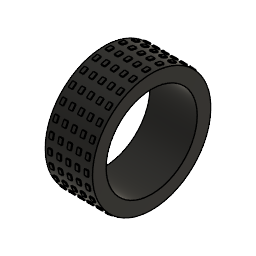
Wheel (Autodesk Fusion 360 archive; units mm, degrees)
design "Piece1"
part number: 2026-01-02-17-32-33-546
Autodesk Fusion 360 part; units mm, degrees
note: some values were not read from the file. Chosen so that the rebuilt part matches the saved one: which bodies a step acts on.
sketch "Boceto1" plane through (0, 0, 0) normal (1, 0, 0) x (0, 1, 0)
  circle A0 centre (0, 0) radius 25
  circle A1 centre (0, 0) radius 32.5
  dimension "d1" = 50
  dimension "d2" = 65
  constraint coincident A0.centre A1.centre
  constraint concentric A0 A1
  measures "d1" diameter of A0
  measures "d2" diameter of A1
extrude "Ancho" add sketch "Boceto1" along normal blind 26 makes body 1
ref_plane "PlanoDeObra1" through (16.1353, 0, 32.5) normal (0, 0, 1) x (0, 1, 0)
sketch "Boceto2" plane through (0, 0, 32.5) normal (0, 0, 1) x (1, 0, 0)
  line L0 (0, 0) -> (13, 0) construction
  line L1 (14, 1.5) -> (12, 1.5)
  line L2 (12, 1.5) -> (12, -1.5)
  line L3 (12, -1.5) -> (14, -1.5)
  line L4 (14, -1.5) -> (14, 1.5)
  line L5 (14, 1.5) -> (12, -1.5) construction
  line L6 (12, 1.5) -> (14, -1.5) construction
  line L7 (13, 0) -> (13, 32.5) construction
  line L8 (4, 1.5) -> (2, 1.5)
  line L9 (2, 1.5) -> (2, -1.5)
  line L10 (4, -1.5) -> (4, 1.5)
  line L11 (2, -1.5) -> (4, -1.5)
  line L12 (9, 1.5) -> (7, 1.5)
  line L13 (7, 1.5) -> (7, -1.5)
  line L14 (9, -1.5) -> (9, 1.5)
  line L15 (7, -1.5) -> (9, -1.5)
  line L16 (19, 1.5) -> (17, 1.5)
  line L17 (17, 1.5) -> (17, -1.5)
  line L18 (19, -1.5) -> (19, 1.5)
  line L19 (17, -1.5) -> (19, -1.5)
  line L20 (24, 1.5) -> (22, 1.5)
  line L21 (22, 1.5) -> (22, -1.5)
  line L22 (24, -1.5) -> (24, 1.5)
  line L23 (22, -1.5) -> (24, -1.5)
  point P0 (13, 0)
  dimension "d6" = 13
  dimension "d7" = 3
  dimension "d8" = 2
  dimension "d9" = 32.5
  dimension "d12" = 10
  dimension "d13" = 0
  constraint coincident L0.start origin
  constraint horizontal L0
  constraint horizontal L1
  constraint perpendicular L1 L2
  constraint parallel L1 L3
  constraint parallel L2 L4
  constraint coincident L5 P0
  constraint coincident L6 P0
  constraint coincident P0 L0.end
  constraint perpendicular L0 L7
  measures "d6" distance of L0.start P0
  measures "d7" distance of L1.end L2.end
  measures "d8" distance of L1.start L1.end
  measures "d9" distance of P0 L7.end
extrude "Altura" add sketch "Boceto2" along normal blind 0.5 separate body makes body 2 at (12.6667, -0.5, 32.5) makes body 3 at (7.6667, -0.5, 32.5) makes body 4 at (18.3333, -0.5, 32.5) makes body 5 at (2.6667, -0.5, 32.5) makes body 6 at (22.6667, -0.5, 32.5)
pattern_circular "Patrón C1" count 28 over 360 about axis through (0, 0, 0) along (1, 0, 0) of bodies 5 3 2 4 6 makes body 7 at (12.6667, -7.7194, 31.5739) makes body 8 at (12.6667, -14.5517, 29.0645) makes body 9 at (12.6667, -20.6543, 25.0978) makes body 10 at (12.6667, -25.7213, 19.8725) makes body 11 at (12.6667, -29.4984, 13.6507) makes body 12 at (12.6667, -31.7964, 6.7445) makes body 13 at (12.6667, -32.5, -0.5) makes body 14 at (12.6667, -31.5739, -7.7194) makes body 15 at (12.6667, -29.0645, -14.5517) makes body 16 at (12.6667, -25.0978, -20.6543) makes body 17 at (12.6667, -19.8725, -25.7213) makes body 18 at (12.6667, -13.6507, -29.4984) makes body 19 at (12.6667, -6.7445, -31.7964) makes body 20 at (12.6667, 0.5, -32.5) makes body 21 at (12.6667, 7.7194, -31.5739) makes body 22 at (12.6667, 14.5517, -29.0645) makes body 23 at (12.6667, 20.6543, -25.0978) makes body 24 at (12.6667, 25.7213, -19.8725) makes body 25 at (12.6667, 29.4984, -13.6507) makes body 26 at (12.6667, 31.7964, -6.7445) makes body 27 at (12.6667, 32.5, 0.5) makes body 28 at (12.6667, 31.5739, 7.7194) makes body 29 at (12.6667, 29.0645, 14.5517) makes body 30 at (12.6667, 25.0978, 20.6543) makes body 31 at (12.6667, 19.8725, 25.7213) makes body 32 at (12.6667, 13.6507, 29.4984) makes body 33 at (12.6667, 6.7445, 31.7964) makes body 34 at (7.6667, -7.7194, 31.5739) makes body 35 at (7.6667, -14.5517, 29.0645) makes body 36 at (7.6667, -20.6543, 25.0978) makes body 37 at (7.6667, -25.7213, 19.8725) makes body 38 at (7.6667, -29.4984, 13.6507) makes body 39 at (7.6667, -31.7964, 6.7445) makes body 40 at (7.6667, -32.5, -0.5) makes body 41 at (7.6667, -31.5739, -7.7194) makes body 42 at (7.6667, -29.0645, -14.5517) makes body 43 at (7.6667, -25.0978, -20.6543) makes body 44 at (7.6667, -19.8725, -25.7213) makes body 45 at (7.6667, -13.6507, -29.4984) makes body 46 at (7.6667, -6.7445, -31.7964) makes body 47 at (7.6667, 0.5, -32.5) makes body 48 at (7.6667, 7.7194, -31.5739) makes body 49 at (7.6667, 14.5517, -29.0645) makes body 50 at (7.6667, 20.6543, -25.0978) makes body 51 at (7.6667, 25.7213, -19.8725) makes body 52 at (7.6667, 29.4984, -13.6507) makes body 53 at (7.6667, 31.7964, -6.7445) makes body 54 at (7.6667, 32.5, 0.5) makes body 55 at (7.6667, 31.5739, 7.7194) makes body 56 at (7.6667, 29.0645, 14.5517) makes body 57 at (7.6667, 25.0978, 20.6543) makes body 58 at (7.6667, 19.8725, 25.7213) makes body 59 at (7.6667, 13.6507, 29.4984) makes body 60 at (7.6667, 6.7445, 31.7964) makes body 61 at (18.3333, -7.7194, 31.5739) makes body 62 at (18.3333, -14.5517, 29.0645) makes body 63 at (18.3333, -20.6543, 25.0978) makes body 64 at (18.3333, -25.7213, 19.8725) makes body 65 at (18.3333, -29.4984, 13.6507) makes body 66 at (18.3333, -31.7964, 6.7445) makes body 67 at (18.3333, -32.5, -0.5) makes body 68 at (18.3333, -31.5739, -7.7194) makes body 69 at (18.3333, -29.0645, -14.5517) makes body 70 at (18.3333, -25.0978, -20.6543) makes body 71 at (18.3333, -19.8725, -25.7213) makes body 72 at (18.3333, -13.6507, -29.4984) makes body 73 at (18.3333, -6.7445, -31.7964) makes body 74 at (18.3333, 0.5, -32.5) makes body 75 at (18.3333, 7.7194, -31.5739) makes body 76 at (18.3333, 14.5517, -29.0645) makes body 77 at (18.3333, 20.6543, -25.0978) makes body 78 at (18.3333, 25.7213, -19.8725) makes body 79 at (18.3333, 29.4984, -13.6507) makes body 80 at (18.3333, 31.7964, -6.7445) makes body 81 at (18.3333, 32.5, 0.5) makes body 82 at (18.3333, 31.5739, 7.7194) makes body 83 at (18.3333, 29.0645, 14.5517) makes body 84 at (18.3333, 25.0978, 20.6543) makes body 85 at (18.3333, 19.8725, 25.7213) makes body 86 at (18.3333, 13.6507, 29.4984) makes body 87 at (18.3333, 6.7445, 31.7964) makes body 88 at (2.6667, -7.7194, 31.5739) makes body 89 at (2.6667, -14.5517, 29.0645) makes body 90 at (2.6667, -20.6543, 25.0978) makes body 91 at (2.6667, -25.7213, 19.8725) makes body 92 at (2.6667, -29.4984, 13.6507) makes body 93 at (2.6667, -31.7964, 6.7445) makes body 94 at (2.6667, -32.5, -0.5) makes body 95 at (2.6667, -31.5739, -7.7194) makes body 96 at (2.6667, -29.0645, -14.5517) makes body 97 at (2.6667, -25.0978, -20.6543) makes body 98 at (2.6667, -19.8725, -25.7213) makes body 99 at (2.6667, -13.6507, -29.4984) makes body 100 at (2.6667, -6.7445, -31.7964) makes body 101 at (2.6667, 0.5, -32.5) makes body 102 at (2.6667, 7.7194, -31.5739) makes body 103 at (2.6667, 14.5517, -29.0645) makes body 104 at (2.6667, 20.6543, -25.0978) makes body 105 at (2.6667, 25.7213, -19.8725) makes body 106 at (2.6667, 29.4984, -13.6507) makes body 107 at (2.6667, 31.7964, -6.7445) makes body 108 at (2.6667, 32.5, 0.5) makes body 109 at (2.6667, 31.5739, 7.7194) makes body 110 at (2.6667, 29.0645, 14.5517) makes body 111 at (2.6667, 25.0978, 20.6543) makes body 112 at (2.6667, 19.8725, 25.7213) makes body 113 at (2.6667, 13.6507, 29.4984) makes body 114 at (2.6667, 6.7445, 31.7964) makes body 115 at (22.6667, -7.7194, 31.5739) makes body 116 at (22.6667, -14.5517, 29.0645) makes body 117 at (22.6667, -20.6543, 25.0978) makes body 118 at (22.6667, -25.7213, 19.8725) makes body 119 at (22.6667, -29.4984, 13.6507) makes body 120 at (22.6667, -31.7964, 6.7445) makes body 121 at (22.6667, -32.5, -0.5) makes body 122 at (22.6667, -31.5739, -7.7194) makes body 123 at (22.6667, -29.0645, -14.5517) makes body 124 at (22.6667, -25.0978, -20.6543) makes body 125 at (22.6667, -19.8725, -25.7213) makes body 126 at (22.6667, -13.6507, -29.4984) makes body 127 at (22.6667, -6.7445, -31.7964) makes body 128 at (22.6667, 0.5, -32.5) makes body 129 at (22.6667, 7.7194, -31.5739) makes body 130 at (22.6667, 14.5517, -29.0645) makes body 131 at (22.6667, 20.6543, -25.0978) makes body 132 at (22.6667, 25.7213, -19.8725) makes body 133 at (22.6667, 29.4984, -13.6507) makes body 134 at (22.6667, 31.7964, -6.7445) makes body 135 at (22.6667, 32.5, 0.5) makes body 136 at (22.6667, 31.5739, 7.7194) makes body 137 at (22.6667, 29.0645, 14.5517) makes body 138 at (22.6667, 25.0978, 20.6543) makes body 139 at (22.6667, 19.8725, 25.7213) makes body 140 at (22.6667, 13.6507, 29.4984) makes body 141 at (22.6667, 6.7445, 31.7964)
combine "Combinar1" operation add target body 1 tool bodies 21 18 26 4 5 10 11 13 7 14 15 6 8 9 12 3 16 17 19 20 22 23 24 25 28 29 30 32 34 35 36 33 38 39 40 41 37 42 27 43 44 45 46 47 48 49 31 55 57 58 59 54 52 53 51 56 50 64 78 80 84 86 88 67 83 92 94 82 97 60 62 68 69 66 61 63 71 65 72 73 74 75 70 76 77 79 81 85 87 89 90 91 93 95 96 99 102 103 104 105 107 100 108 109 110 111 101 98 112 113 114 106 121 115 122 116 118 120 119 123 117 124 128 140 130 132 134 136 139 126 141 135 138 127 125 129 133 137 131 2
equation "d6 = ( 26 / 2 ) * 1 mm"
equation "d9 = ( 65 / 2 ) * 1 mm"
named bodies: "Llanta"

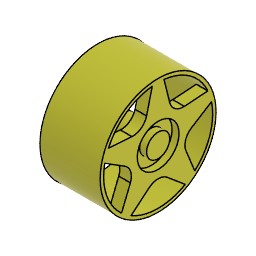
design "Piece2"
part number: 2026-01-02-23-41-02-488
Autodesk Fusion 360 part; units mm, degrees
sketch "Boceto1" plane through (0, 0, 0) normal (1, 0, 0) x (0, 1, 0)
  circle A0 centre (0, 0) radius 25
  dimension "d1" = 50
  constraint coincident A0.centre origin
  measures "d1" diameter of A0
extrude "Extruir1" add sketch "Boceto1" along normal blind 26
sketch "Boceto2" plane through (26, 0, 0) normal (1, 0, 0) x (0, 1, 0)
  circle A0 centre (0, 0) radius 25
  circle A1 centre (0, 0) radius 5
  circle A2 centre (0, 0) radius 9
  dimension "d4" = 10
  dimension "d5" = 18
  constraint coincident A0.centre A1.centre
  measures "d4" diameter of A1
  measures "d5" diameter of A2
extrude "Extruir2" cut sketch "Boceto2" against normal blind 3 contours A2
sketch "Boceto3" plane through (26, 0, 0) normal (1, 0, 0) x (0, 1, 0)
  circle A0 centre (0, 0) radius 25
  circle A1 centre (0, 0) radius 9
  circle A2 centre (0, 0) radius 23.5
  line L0 (0, 23.5) -> (0, 13.5) construction
  line L1 (0, 13.5) -> (-5, 13.5)
  line L2 (0, 13.5) -> (5, 13.5)
  line L3 (0, 23.5) -> (-2.5, 23.5)
  line L4 (-2.5, 23.5) -> (-5, 13.5)
  line L5 (2.5, 23.5) -> (5, 13.5)
  line L6 (0, 23.5) -> (2.5, 23.5)
  line L7 (-12.8393, 4.1717) -> (-11.2942, 8.927)
  line L8 (-12.8393, 4.1717) -> (-14.3843, -0.5836)
  line L9 (-23.1224, 4.8843) -> (-14.3843, -0.5836)
  line L10 (-22.3498, 7.2619) -> (-23.1224, 4.8843)
  line L11 (-22.3498, 7.2619) -> (-21.5773, 9.6395)
  line L12 (-21.5773, 9.6395) -> (-11.2942, 8.927)
  line L13 (-7.9351, -10.9217) -> (-11.9802, -7.9828)
  line L14 (-7.9351, -10.9217) -> (-3.89, -13.8607)
  line L15 (-11.7904, -20.4814) -> (-3.89, -13.8607)
  line L16 (-13.813, -19.0119) -> (-11.7904, -20.4814)
  line L17 (-13.813, -19.0119) -> (-15.8355, -17.5424)
  line L18 (-15.8355, -17.5424) -> (-11.9802, -7.9828)
  line L19 (7.9351, -10.9217) -> (3.89, -13.8607)
  line L20 (7.9351, -10.9217) -> (11.9802, -7.9828)
  line L21 (15.8355, -17.5424) -> (11.9802, -7.9828)
  line L22 (13.813, -19.0119) -> (15.8355, -17.5424)
  line L23 (13.813, -19.0119) -> (11.7904, -20.4814)
  line L24 (11.7904, -20.4814) -> (3.89, -13.8607)
  line L25 (12.8393, 4.1717) -> (14.3843, -0.5836)
  line L26 (12.8393, 4.1717) -> (11.2942, 8.927)
  line L27 (21.5773, 9.6395) -> (11.2942, 8.927)
  line L28 (22.3498, 7.2619) -> (21.5773, 9.6395)
  line L29 (22.3498, 7.2619) -> (23.1224, 4.8843)
  line L30 (23.1224, 4.8843) -> (14.3843, -0.5836)
  arc A3 (-11.2942, 8.927) -> (-5, 13.5) centre (-10.8755, 14.9689) ccw
  arc A4 (-11.9802, -7.9828) -> (-14.3843, -0.5836) centre (-17.597, -5.7176) ccw
  arc A5 (3.89, -13.8607) -> (-3.89, -13.8607) centre (0, -18.5026) ccw
  arc A6 (14.3843, -0.5836) -> (11.9802, -7.9828) centre (17.597, -5.7176) ccw
  arc A7 (5, 13.5) -> (11.2942, 8.927) centre (10.8755, 14.9689) ccw
  dimension "d8" = 47
  dimension "d9" = 10
  dimension "d10" = 5
  dimension "d12" = 2.5
  dimension "d14" = 360
  constraint coincident A0.centre A1.centre
  constraint coincident A2 L0.start
  constraint vertical L0
  constraint perpendicular L0 L1
  constraint symmetric L1.start L0 L2.start
  constraint symmetric L0 L1.end L2.end
  constraint perpendicular L0 L3
  constraint symmetric L3.start L0 L6.start
  constraint symmetric L0 L3.end L5.start
  constraint tangent L4 A3
  constraint tangent L9 A4
  constraint tangent L15 A5
  constraint tangent L21 A6
  constraint tangent L27 A7
  measures "d8" diameter of A2
  measures "d9" distance of L0.start L0.end
  measures "d10" distance of L0.end L1.end
  measures "d12" distance of L0.start L3.end
extrude "Extruir3" cut sketch "Boceto3" against normal through all contours A2 L21 L30 A6 | A2 L5 L27 A7 | A2 L15 L24 A5 | A2 L4 L12 A3 | A2 L9 L18 A4
sketch "Boceto4" plane through (0, 0, 0) normal (-1, 0, 0) x (0, -1, 0)
  line L0 (-11.9802, -7.9828) -> (-15.7827, -17.4114)
  arc A0 (-23.0026, 4.8093) -> (-15.7827, -17.4114) centre (0, 0) ccw
  line L1 (-23.0026, 4.8093) -> (-14.3843, -0.5836)
  arc A1 (-11.9802, -7.9828) -> (-14.3843, -0.5836) centre (-17.597, -5.7176) ccw
  line L2 (-11.2942, 8.927) -> (-21.4364, 9.6298)
  arc A2 (-2.5343, 23.363) -> (-21.4364, 9.6298) centre (0, 0) ccw
  line L3 (-2.5343, 23.363) -> (-5, 13.5)
  arc A3 (-11.2942, 8.927) -> (-5, 13.5) centre (-10.8755, 14.9689) ccw
  line L4 (3.89, -13.8607) -> (11.6821, -20.3906)
  arc A4 (-11.6821, -20.3906) -> (11.6821, -20.3906) centre (0, 0) ccw
  line L5 (-11.6821, -20.3906) -> (-3.89, -13.8607)
  arc A5 (3.89, -13.8607) -> (-3.89, -13.8607) centre (0, -18.5026) ccw
  line L6 (5, 13.5) -> (2.5343, 23.363)
  arc A6 (21.4364, 9.6298) -> (2.5343, 23.363) centre (0, 0) ccw
  line L7 (21.4364, 9.6298) -> (11.2942, 8.927)
  arc A7 (5, 13.5) -> (11.2942, 8.927) centre (10.8755, 14.9689) ccw
  line L8 (14.3843, -0.5836) -> (23.0026, 4.8093)
  arc A8 (15.7827, -17.4114) -> (23.0026, 4.8093) centre (0, 0) ccw
  line L9 (15.7827, -17.4114) -> (11.9802, -7.9828)
  arc A9 (14.3843, -0.5836) -> (11.9802, -7.9828) centre (17.597, -5.7176) ccw
  circle A10 centre (0, 0) radius 25
  circle A11 centre (0, 0) radius 23.5
  constraint coincident A0.centre A2.centre
extrude "Extruir4" cut sketch "Boceto4" against normal blind 21 contours L0 L1 A1 L2 L3 A3 L4 L5 A5 L6 L7 A7 L8 L9 A9 A11
sketch "Boceto5" plane through (21, 0, 0) normal (-1, 0, 0) x (0, -1, 0)
  line L0 (3.89, -13.8607) -> (11.6821, -20.3906)
  arc A0 (11.6821, -20.3906) -> (15.7827, -17.4114) centre (0, 0) ccw
  line L1 (15.7827, -17.4114) -> (11.9802, -7.9828)
  arc A1 (14.3843, -0.5836) -> (11.9802, -7.9828) centre (17.597, -5.7176) ccw
  line L2 (14.3843, -0.5836) -> (23.0026, 4.8093)
  arc A2 (23.0026, 4.8093) -> (21.4364, 9.6298) centre (0, 0) ccw
  line L3 (21.4364, 9.6298) -> (11.2942, 8.927)
  arc A3 (5, 13.5) -> (11.2942, 8.927) centre (10.8755, 14.9689) ccw
  line L4 (5, 13.5) -> (2.5343, 23.363)
  arc A4 (2.5343, 23.363) -> (-2.5343, 23.363) centre (0, 0) ccw
  line L5 (-2.5343, 23.363) -> (-5, 13.5)
  arc A5 (-11.2942, 8.927) -> (-5, 13.5) centre (-10.8755, 14.9689) ccw
  line L6 (-11.2942, 8.927) -> (-21.4364, 9.6298)
  arc A6 (-21.4364, 9.6298) -> (-23.0026, 4.8093) centre (0, 0) ccw
  line L7 (-23.0026, 4.8093) -> (-14.3843, -0.5836)
  arc A7 (-11.9802, -7.9828) -> (-14.3843, -0.5836) centre (-17.597, -5.7176) ccw
  line L8 (-11.9802, -7.9828) -> (-15.7827, -17.4114)
  arc A8 (-15.7827, -17.4114) -> (-11.6821, -20.3906) centre (0, 0) ccw
  line L9 (-11.6821, -20.3906) -> (-3.89, -13.8607)
  arc A9 (3.89, -13.8607) -> (-3.89, -13.8607) centre (0, -18.5026) ccw
  circle A10 centre (0, 0) radius 5
  dimension "d18" = 10
  constraint coincident A0.centre A2.centre
  measures "d18" diameter of A10
extrude "Extruir5" add sketch "Boceto5" along normal blind 10 contours A10
sketch "Boceto6" plane through (11, 0, 0) normal (-1, 0, 0) x (0, -1, 0)
  circle A0 centre (0, 0) radius 5
  line L0 (1.85, 1.9666) -> (-1.85, 1.9666)
  line L1 (-1.85, -1.9666) -> (1.85, -1.9666)
  arc A1 (-1.85, 1.9666) -> (-1.85, -1.9666) centre (0, 0) ccw
  arc A2 (1.85, -1.9666) -> (1.85, 1.9666) centre (0, 0) ccw
  dimension "d21" = 5.4
  dimension "d22" = 3.7
  constraint coincident A0.centre A1.centre
  constraint horizontal L0
  constraint parallel L0 L1
  constraint concentric A1 A2
  measures "d21" diameter of A1
  measures "d22" distance of L0.start L0.end
extrude "Extruir6" cut sketch "Boceto6" against normal blind 9 contours L0 L1 A1 A2
